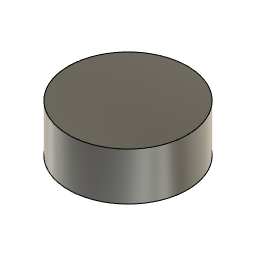
rain (Autodesk Fusion 360 archive; units mm, degrees)
design "magnes"
Autodesk Fusion 360 part; units mm, degrees
note: some values were not read from the file. Set by a fixed rule: which face or edge a step refers to.
sketch "Szkic1" plane through (0, 0, 0) normal (0, 0, 1) x (1, 0, 0)
  circle A0 centre (0, 0) radius 5
  dimension "d1" = 10
  constraint coincident A0.centre origin
  measures "d1" diameter of A0
extrude "Wyciągnięcie proste1" add sketch "Szkic1" along normal blind 4

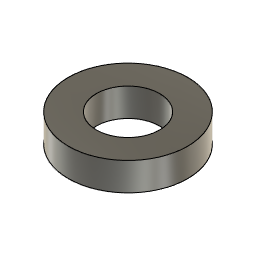
design "lozysko"
Autodesk Fusion 360 part; units mm, degrees
sketch "Szkic1" plane through (0, 0, 0) normal (0, 0, 1) x (1, 0, 0)
  circle A0 centre (0, 0) radius 4.5
  circle A1 centre (0, 0) radius 8.5
  dimension "d1" = 9
  dimension "d2" = 17
  constraint coincident A0.centre A1.centre
  constraint concentric A0 A1
  measures "d1" diameter of A0
  measures "d2" diameter of A1
extrude "Wyciągnięcie proste1" add sketch "Szkic1" along normal blind 4

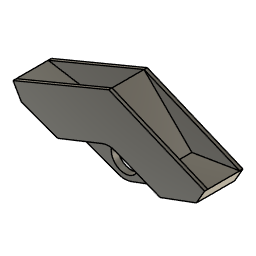
design "baseny"
Autodesk Fusion 360 part; units mm, degrees
sketch "Sketch1" plane through (0, 0, 0) normal (0, 1, 0) x (1, 0, 0)
  line L0 (-30, 0) -> (0, -30)
  line L1 (0, 0) -> (-30, 0)
  line L2 (0, 0) -> (0, -55)
  line L3 (-30, 0) -> (-60, -5)
  circle A0 centre (0, 12) radius 4.5
  circle A1 centre (0, 12) radius 8.55
  line L4 (-60, -5) -> (-54.8038, 4)
  line L5 (-60, -5) -> (-60.4903, -5) construction
  line L6 (-54.8038, 4) -> (-3.9877, 22.7865)
  line L7 (60, -5) -> (54.8038, 4)
  line L8 (30, 0) -> (60, -5)
  line L9 (30, 0) -> (0, -30)
  line L10 (-60, -5) -> (0, -30)
  line L11 (60, -5) -> (0, -30)
  circle A2 centre (0, 12) radius 11.5
  line L12 (-32.1229, 12.385) -> (-4.2451, 1.3122)
  line L13 (32.1229, 12.385) -> (4.2451, 1.3122)
  line L14 (54.8038, 4) -> (3.9877, 22.7865)
  dimension "d3" = 30
  dimension "d4" = 30
  dimension "d6" = 30
  dimension "d7" = 5
  dimension "d8" = 9
  dimension "d9" = 17.1
  dimension "d10" = 60
  dimension "d11" = 12
  dimension "d12" = 23
  dimension "d31" = 4
  constraint coincident L1.start L2.start
  constraint horizontal L1
  constraint perpendicular L1 L2
  constraint coincident L0.end L2
  constraint concentric A0 A1
  constraint horizontal L5
  constraint symmetric L0.start L2 L8.start
  constraint symmetric L0.end L2 L9.end
  constraint symmetric L2 L3.end L7.start
  constraint symmetric L2 L7.end L4.end
  constraint coincident L2 A0.centre
  constraint symmetric L2 L0.end L9.end
  constraint concentric A0 A2
  constraint tangent L6 A2
  constraint coincident L6.end A2
  constraint coincident L6 L12.start
  constraint coincident A2 L12.end
  constraint tangent A2 L12
  constraint symmetric L2 L6.end L14.end
  constraint symmetric L2 L12.start L13.start
  constraint symmetric L2 L12.end L13.end
  constraint symmetric L2 L4.end L7.end
  measures "d3" distance of L1.start L0.end
  measures "d4" distance of L1.start L0.start
  measures "d6" horizontal distance of L0.start L3.end
  measures "d7" vertical distance of L0.start L3.end
  measures "d8" diameter of A0
  measures "d9" diameter of A1
  measures "d10" angle of L4 L5
  measures "d11" distance of L1.start A0.centre
  measures "d12" diameter of A2
  measures "d31" vertical distance of L0.start L4.end
extrude "Extrude1" add sketch "Sketch1" along normal mid plane 24 contours L0 L1 L2 | L1 L2 L3 L4 L6 L7 L8 L9 A2 L12 L13 L14 | L0 L3 L10 | L8 L9 L11
extrude "Extrude2" cut sketch "Sketch1" along normal mid plane 20 contours L0 L3 L10 | L8 L9 L11
extrude "Extrude3" add sketch "Sketch1" along normal mid plane 4 contours L6 A2 L12 | A2 L13 L14 | A2
sketch "Sketch2" plane through (-7.8906, 0, -21.3436) normal (-0.346757, 0, -0.937955) x (0, -1, 0)
  line L0 (2, 25.8353) -> (12, 25.8353)
  line L1 (12, 25.8353) -> (12, 50.0165)
  line L2 (12, 50.0165) -> (-12, 50.0165)
  line L3 (-12, 50.0165) -> (-12, 25.8353)
  line L4 (-12, 25.8353) -> (-2, 25.8353)
  line L5 (-2, 25.8353) -> (-2, -4.1611)
  line L6 (-2, -4.1611) -> (2, -4.1611)
  line L7 (2, -4.1611) -> (2, 25.8353)
  circle A0 centre (0, 33.8389) radius 5
  circle A1 centre (0, 33.8389) radius 7
  circle A2 centre (0, 42.8389) radius 2.05
  circle A3 centre (0, 24.8389) radius 2.05
  circle A4 centre (0, 42.8389) radius 3
  circle A5 centre (0, 24.8389) radius 3
  dimension "d19" = 10
  dimension "d20" = 14
  dimension "d21" = 4.1
  dimension "d22" = 9
  dimension "d23" = 4.1
  dimension "d24" = 9
  dimension "d25" = 6
  dimension "d26" = 6
  dimension "d40" = 38
  constraint concentric A0 A1
  constraint concentric A2 A4
  constraint concentric A3 A5
  measures "d19" diameter of A0
  measures "d20" diameter of A1
  measures "d21" diameter of A2
  measures "d22" distance of A0.centre A2.centre
  measures "d23" diameter of A3
  measures "d24" distance of A0.centre A3.centre
  measures "d25" diameter of A4
  measures "d26" diameter of A5
  measures "d40" distance of L6 A0.centre
extrude "Extrude6" add sketch "Sketch2" along normal up to surface contours L0 L7 A3 A5 | L7 A3 | L5 A3 | L4 L5 A3 A5 end surface through (-32.1229, 0, -12.385) normal (0.369139, 0, -0.929374) offset 0
extrude "Extrude11" cut sketch "Sketch2" against normal blind 7 contours L7 A3 | L5 L7 A1 A3 | A1 A3 | L5 A3 | A1 A2 | A1 A2
sketch "Sketch4" plane through (7.8906, 0, -21.3436) normal (0.346757, 0, -0.937955) x (0, 1, 0)
  line L0 (12, 50.0165) -> (-12, 50.0165)
  line L1 (-12, 50.0165) -> (-12, 25.8353)
  line L2 (-12, 25.8353) -> (-2, 25.8353)
  line L3 (-2, 25.8353) -> (-2, -4.1611)
  line L4 (-2, -4.1611) -> (2, -4.1611)
  line L5 (2, -4.1611) -> (2, 25.8353)
  line L6 (2, 25.8353) -> (12, 25.8353)
  line L7 (12, 25.8353) -> (12, 50.0165)
  circle A0 centre (0, 33.8389) radius 5
  circle A1 centre (0, 33.8389) radius 7
  circle A2 centre (0, 24.8389) radius 2.05
  circle A3 centre (0, 24.8389) radius 3
  circle A4 centre (0, 42.8389) radius 2.05
  circle A5 centre (0, 42.8389) radius 3
  dimension "d44" = 10
  dimension "d45" = 14
  dimension "d46" = 4.1
  dimension "d47" = 6
  dimension "d48" = 9
  dimension "d49" = 4.1
  dimension "d50" = 6
  dimension "d51" = 9
  dimension "d59" = 38
  constraint concentric A0 A1
  constraint concentric A2 A3
  constraint concentric A4 A5
  measures "d44" diameter of A0
  measures "d45" diameter of A1
  measures "d46" diameter of A2
  measures "d47" diameter of A3
  measures "d48" distance of A0.centre A2.centre
  measures "d49" diameter of A4
  measures "d50" diameter of A5
  measures "d51" distance of A0.centre A4.centre
  measures "d59" distance of L4 A0.centre
extrude "Extrude8" add sketch "Sketch4" along normal up to surface contours L5 L6 A2 A3 | L2 L3 A2 A3 | L5 A2 | L3 A2 end surface through (32.1229, 0, -12.385) normal (-0.369139, 0, -0.929374) offset 0
extrude "Extrude10" cut sketch "Sketch4" against normal blind 7 contours L5 A2 | L3 L5 A1 A2 | A1 A2 | L3 A2 | A1 A4 | A1 A4

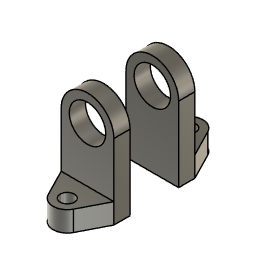
design "mocowanie sworzen"
Autodesk Fusion 360 part; units mm, degrees
sketch "Sketch1" plane through (0, 0, 0) normal (0, 0, 1) x (1, 0, 0)
  line L0 (6.5, 10) -> (-6.5, 10)
  line L1 (-6.5, 10) -> (-6.5, -10)
  line L2 (-6.5, -10) -> (6.5, -10)
  line L3 (6.5, -10) -> (6.5, 10)
  line L4 (6.5, 10) -> (-6.5, -10) construction
  line L5 (-6.5, 10) -> (6.5, -10) construction
  line L6 (-6.5, 10) -> (6.5, 10)
  line L7 (6.5, 10) -> (6.5, 6)
  line L8 (6.5, 6) -> (-6.5, 6)
  line L9 (-6.5, 6) -> (-6.5, 10)
  line L10 (-6.5, -10) -> (6.5, -10)
  line L11 (6.5, -10) -> (6.5, -6)
  line L12 (6.5, -6) -> (-6.5, -6)
  line L13 (-6.5, -6) -> (-6.5, -10)
  circle A0 centre (0, 15) radius 1.75
  circle A1 centre (0, -15) radius 1.75
  circle A2 centre (0, 15) radius 3.5
  circle A3 centre (0, -15) radius 3.5
  line L14 (-6.5, 10) -> (-3.1139, 16.598)
  line L15 (6.5, 10) -> (3.1139, 16.598)
  line L16 (-6.5, -10) -> (-3.1139, -16.598)
  line L17 (6.5, -10) -> (3.1139, -16.598)
  dimension "d1" = 13
  dimension "d2" = 20
  dimension "d3" = 4
  dimension "d4" = 4
  dimension "d5" = 3.5
  dimension "d6" = 15
  dimension "d7" = 3.5
  dimension "d8" = 15
  dimension "d9" = 7
  dimension "d10" = 7
  constraint horizontal L0
  constraint perpendicular L0 L1
  constraint parallel L0 L2
  constraint parallel L1 L3
  constraint coincident L4 origin
  constraint coincident L5 origin
  constraint horizontal L6
  constraint vertical L7
  constraint horizontal L8
  constraint vertical L9
  constraint coincident L3 L7.end
  constraint horizontal L10
  constraint vertical L11
  constraint horizontal L12
  constraint vertical L13
  constraint concentric A0 A2
  constraint concentric A1 A3
  constraint coincident A2 L14.end
  constraint tangent A2 L14
  constraint coincident A2 L15.end
  constraint tangent A2 L15
  constraint coincident A3 L16.end
  constraint tangent A3 L16
  constraint coincident A3 L17.end
  constraint tangent A3 L17
  constraint vertical origin A1.centre
  constraint vertical origin A0.centre
  measures "d1" distance of L1.end L2.end
  measures "d2" distance of L0.end L1.end
  measures "d3" distance of L0.end L8.end
  measures "d4" distance of L1.end L12.end
  measures "d5" diameter of A0
  measures "d6" distance of origin A0.centre
  measures "d7" diameter of A1
  measures "d8" distance of origin A1.centre
  measures "d9" diameter of A2
  measures "d10" diameter of A3
extrude "Extrude1" add sketch "Sketch1" along normal blind 5 contours L0 L1 L3 L6 L7 L8 L9 | L0 L6 A2 L14 L15 | A2 | L1 L2 L3 L10 L11 L12 L13 | L2 L10 A3 L16 L17 | A3 makes body 1 at (0.0436, 8.4183, 0) makes body 2 at (-0.0436, -8.4183, 0)
extrude "Extrude2" add sketch "Sketch1" along normal blind 25 contours L0 L1 L3 L6 L7 L8 L9 | L1 L2 L3 L10 L11 L12 L13 bodies 1 2
sketch "Sketch3" plane through (0, -10, 0) normal (0, -1, 0) x (1, 0, 0)
  line L0 (6.5, 5) -> (6.5, 25)
  line L1 (6.5, 25) -> (-6.5, 25)
  line L2 (-6.5, 25) -> (-6.5, 5)
  circle A0 centre (0, 18.5) radius 4.5
  circle A1 centre (0, 18.5) radius 6.5
  line L3 (-6.5, 5) -> (6.5, 5)
  dimension "d15" = 9
  dimension "d16" = 6.5
  constraint concentric A0 A1
  constraint tangent L0 A1
  measures "d15" diameter of A0
  measures "d16" distance of L1 A0.centre
extrude "Extrude4" cut sketch "Sketch3" against normal blind 20 contours L0 L1 A1 | L1 L2 A1 | A0 bodies 1 2

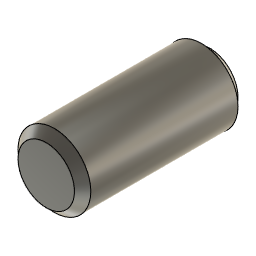
design "sworzen"
Autodesk Fusion 360 part; units mm, degrees
sketch "Sketch1" plane through (0, 0, 0) normal (0, 1, 0) x (1, 0, 0)
  circle A0 centre (0, 0) radius 4.45
  dimension "d1" = 8.9
  constraint coincident A0.centre origin
  measures "d1" diameter of A0
extrude "Extrude1" add sketch "Sketch1" along normal blind 20
chamfer "Chamfer1" distance 1 angle 45 2 edges at (-4.1489, 0, 1.6092) (-4.1489, 20, 1.6092)

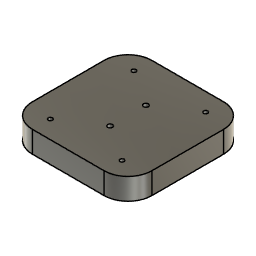
design "obudowa"
Autodesk Fusion 360 part; units mm, degrees
sketch "Sketch1" plane through (0, 0, 0) normal (0, 0, 1) x (1, 0, 0)
  line L0 (50, 50) -> (-50, 50)
  line L1 (-50, 50) -> (-50, -50)
  line L2 (-50, -50) -> (50, -50)
  line L3 (50, -50) -> (50, 50)
  line L4 (50, 50) -> (-50, -50) construction
  line L5 (-50, 50) -> (50, -50) construction
  circle A0 centre (0, 15) radius 2.05
  circle A1 centre (0, -15) radius 2.05
  circle A2 centre (0, 15) radius 4
  circle A3 centre (0, -15) radius 4
  circle A4 centre (30, -35) radius 1.75
  circle A5 centre (30, 35) radius 1.75
  line L6 (0, 0) -> (0, 5)
  circle A6 centre (-30, 35) radius 1.75
  circle A7 centre (-30, -35) radius 1.75
  dimension "d1" = 100
  dimension "d2" = 100
  dimension "d4" = 4.1
  dimension "d5" = 15
  dimension "d6" = 15
  dimension "d8" = 8
  dimension "d36" = 3.5
  dimension "d37" = 3.5
  dimension "d55" = 30
  dimension "d56" = 35
  dimension "d57" = 35
  dimension "d58" = 30
  constraint horizontal L0
  constraint perpendicular L0 L1
  constraint parallel L0 L2
  constraint parallel L1 L3
  constraint coincident L4 L6.start
  constraint coincident L5 L6.start
  constraint coincident L6.start origin
  constraint concentric A0 A2
  constraint concentric A1 A3
  constraint vertical L6
  constraint symmetric A4 L6 A7
  constraint symmetric A5 L6 A6
  constraint equal A0 A1
  constraint equal A2 A3
  constraint vertical L6.start A1.centre
  constraint vertical L6.start A0.centre
  measures "d1" distance of L1.end L2.end
  measures "d2" distance of L0.end L1.end
  measures "d4" diameter of A1
  measures "d5" distance of L6.start A0.centre
  measures "d6" distance of L6.start A1.centre
  measures "d8" diameter of A3
  measures "d36" diameter of A4
  measures "d37" diameter of A5
  measures "d55" horizontal distance of L6.start A5.centre
  measures "d56" vertical distance of L6.start A5.centre
  measures "d57" vertical distance of L6.start A4.centre
  measures "d58" horizontal distance of L6.start A4.centre
extrude "Extrude1" add sketch "Sketch1" along normal blind 3 contours L0 L1 L2 L3 | A2 | A3
extrude "Extrude2" add sketch "Sketch1" against normal blind 5 contours A2 | A3
sketch "Sketch2" plane through (0, 0, -5) normal (0, 0, -1) x (1, 0, 0)
  circle A0 centre (0, 15) radius 2.05
  circle A1 centre (0, 15) radius 4
  circle A2 centre (0, 15) radius 3
  circle A3 centre (0, -15) radius 4
  dimension "d40" = 8
  constraint concentric A0 A2
  measures "d40" diameter of A3
extrude "Extrude3" add sketch "Sketch2" along normal blind 2 contours A0 | A1 | A2 | A3
sketch "Sketch3" plane through (0, 0, 0) normal (0, 0, -1) x (1, 0, 0)
  circle A0 centre (0, -15) radius 4
  circle A1 centre (0, 15) radius 4
  line L0 (50, -50) -> (50, 50)
  line L1 (50, 50) -> (-50, 50)
  line L2 (-50, 50) -> (-50, -50)
  line L3 (-50, -50) -> (50, -50)
  circle A2 centre (30, 35) radius 1.75
  circle A3 centre (30, -35) radius 1.75
  line L4 (-47, 42) -> (47, 42)
  line L5 (47, 42) -> (47, -42)
  line L6 (47, -42) -> (-47, -42)
  line L7 (-47, -42) -> (-47, 42)
  circle A4 centre (-30, 35) radius 1.75
  circle A5 centre (-30, -35) radius 1.75
  dimension "d41" = 3
  dimension "d42" = 3
  dimension "d43" = 8
  dimension "d44" = 8
  constraint horizontal L4
  constraint vertical L5
  constraint horizontal L6
  constraint vertical L7
  measures "d41" distance of L0 L5
  measures "d42" distance of L2 L7
  measures "d43" distance of L3 L6
  measures "d44" distance of L1 L4
extrude "Extrude4" add sketch "Sketch3" along normal blind 15 contours L0 L1 L2 L3
sketch "Sketch6" plane through (0, 0, -15) normal (0, 0, -1) x (1, 0, 0)
  line L0 (47, -42) -> (-47, -42)
  line L1 (-47, -42) -> (-47, 42)
  line L2 (-47, 42) -> (47, 42)
  line L3 (47, 42) -> (47, -42)
  line L4 (-50, -50) -> (50, -50)
  line L5 (50, -50) -> (50, 50)
  line L6 (50, 50) -> (-50, 50)
  line L7 (-50, 50) -> (-50, -50)
  line L8 (0, 0) -> (20, 0)
  circle A0 centre (10, 46) radius 2.05
  line L9 (0, 0) -> (0, 5)
  circle A1 centre (-10, 46) radius 2.05
  circle A2 centre (10, -46) radius 2.05
  circle A3 centre (-10, -46) radius 2.05
  dimension "d45" = 4.1
  dimension "d61" = 4
  dimension "d62" = 10
  constraint coincident L8.start L9.start
  constraint parallel L2 L8
  constraint perpendicular L8 L9
  constraint symmetric A0 L9 A1
  constraint symmetric L8 A0 A2
  constraint symmetric L8 A1 A3
  measures "d45" diameter of A0
  measures "d61" distance of L6 A0.centre
  measures "d62" distance of A0.centre L9
extrude "Extrude7" cut sketch "Sketch6" against normal blind 10 contours A0 | A1 | A2 | A3
fillet "Fillet3" radius 20 8 edges at (47, -42, -7.5) (47, 42, -7.5) (-47, -42, -7.5) (50, -50, -6) (-50, -50, -6) (-50, 50, -6) (-47, 42, -7.5) (50, 50, -6)

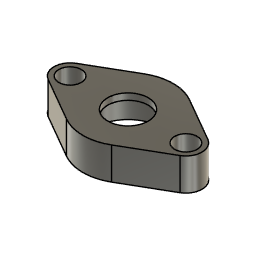
design "uchwyt magnes"
Autodesk Fusion 360 part; units mm, degrees
sketch "Sketch1" plane through (0, 0, 0) normal (0, 0, 1) x (1, 0, 0)
  circle A0 centre (0, 0) radius 5.15
  circle A1 centre (0, 0) radius 7
  circle A2 centre (9, 0) radius 2.5
  circle A3 centre (-9, 0) radius 2.5
  circle A4 centre (-9, 0) radius 1.75
  circle A5 centre (9, 0) radius 1.75
  line L0 (-10.25, 2.1651) -> (-3.5, 6.0622)
  line L1 (-9, 0) -> (9, 0)
  line L2 (-10.25, -2.1651) -> (-3.5, -6.0622)
  line L3 (0, 12) -> (0, 15)
  line L4 (10.25, 2.1651) -> (3.5, 6.0622)
  line L5 (10.25, -2.1651) -> (3.5, -6.0622)
  dimension "d1" = 10.3
  dimension "d2" = 14
  dimension "d3" = 5
  dimension "d4" = 5
  dimension "d5" = 9
  dimension "d6" = 9
  dimension "d7" = 3.5
  dimension "d8" = 3.5
  constraint coincident A0.centre A1.centre
  constraint concentric A0 A1
  constraint concentric A3 A4
  constraint concentric A2 A5
  constraint tangent A1 L0
  constraint coincident A3.centre A4.centre
  constraint coincident A2.centre A5.centre
  constraint horizontal L1
  constraint tangent A3 L0
  constraint tangent A1 L2
  constraint tangent A3 L2
  constraint coincident A1 L0.end
  constraint coincident A1 L2.end
  constraint coincident A3 L2.start
  constraint coincident A3 L0.start
  constraint vertical L3
  constraint symmetric L0.end L3 L4.end
  constraint symmetric L2.end L3 L5.end
  constraint symmetric L2.start L3 L5.start
  constraint symmetric L0.start L3 L4.start
  constraint coincident A1 L5.end
  measures "d1" diameter of A0
  measures "d2" diameter of A1
  measures "d3" diameter of A2
  measures "d4" diameter of A3
  measures "d5" distance of A0.centre A3.centre
  measures "d6" distance of A0.centre A2.centre
  measures "d7" diameter of A4
  measures "d8" diameter of A5
extrude "Extrude1" add sketch "Sketch1" along normal blind 5 contours A0 A1 A2 A3 L1 | A0 A1 A2 A3 L1 | A1 A2 L1 | A1 A2 L1 | A1 A3 L1 | A1 A3 L1 | A1 A2 | A1 A2 L4 | A1 A2 L5 | A1 A3 L0 | A1 A3 | A1 A3 L2
sketch "Sketch2" plane through (0, 0, 5) normal (0, 0, 1) x (-1, 0, 0)
  circle A0 centre (-9, 0) radius 1.75
  circle A1 centre (0, 0) radius 5.15
  circle A2 centre (9, 0) radius 1.75
  line L0 (-10.25, -2.1651) -> (-3.5, -6.0622)
  arc A3 (-3.5, -6.0622) -> (3.5, -6.0622) centre (0, 0) ccw
  line L1 (3.5, -6.0622) -> (10.25, -2.1651)
  arc A4 (10.25, -2.1651) -> (10.25, 2.1651) centre (9, 0) ccw
  line L2 (10.25, 2.1651) -> (3.5, 6.0622)
  arc A5 (3.5, 6.0622) -> (-3.5, 6.0622) centre (0, 0) ccw
  line L3 (-3.5, 6.0622) -> (-10.25, 2.1651)
  arc A6 (-10.25, 2.1651) -> (-10.25, -2.1651) centre (-9, 0) ccw
  circle A7 centre (0, 0) radius 3.15
  dimension "d11" = -2
extrude "Extrude2" add sketch "Sketch2" against normal blind 1 contours A1
